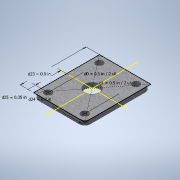
# Autodesk Inventor part: J010354
Saved by Autodesk Inventor 2020.3 (Build 243373000, 373)
## iProperties
RuleStatus: InUse
AfterDocSave0: file://Part Number Cleaner
Created: 2022-03-31
Material: STAINLESS STEEL, 304
Catalog Web Link: https://www.janelia.org/
Vendor: HHMI: JRC - jET
Document SubType Name: Modeling
Designer: arnoldj
Density: 8 g/cm^3
Appearance: Metal-Steel (Stainless, Brushed)
Part Number: J010354
Description: FB CYLINDER PLATE
DESIGN DEPARTMENT: HHMI: JRC - jET
ALTERED ITEM PART NUMBER: N/A
ALTERED ITEM VENDOR: N/A
ALTERED ITEM DESCRIPTION: N/A
Title: Standard
Author: arnoldj
Revision Number: 0
Autodesk Inventor part; units mm, degrees
ref_plane "YZ Plane" through (0, 0, 0) normal (1, 0, 0) x (0, 1, 0)
ref_plane "XZ Plane" through (0, 0, 0) normal (0, 1, 0) x (-1, 0, 0)
ref_plane "XY Plane" through (0, 0, 0) normal (0, 0, 1) x (1, 0, 0)
sketch "Sketch1" plane through (0, 0, 0) normal (0, 1, 0) x (-1, 0, 0)
  line L0 (0, -16.002) -> (0, 16.002) projected
  line L1 (-12.446, 0) -> (12.446, 0) projected
  line L2 (-8.89, 11.43) -> (8.89, 11.43)
  line L3 (8.89, 11.43) -> (8.89, -11.43)
  line L4 (8.89, -11.43) -> (-8.89, -11.43)
  line L5 (-8.89, -11.43) -> (-8.89, 11.43)
  line L6 (-8.89, 11.43) -> (8.89, -11.43) construction
  line L7 (8.89, 11.43) -> (-8.89, -11.43) construction
  point P0 (0, 0)
  point P1 (6.35, 8.89)
  point P2 (-6.35, 8.89)
  dimension "d0" = 6.35
  dimension "d1" = 6.35
  dimension "d23" = 22.86
  dimension "d24" = 17.78
  dimension "d25" = 8.89
  constraints: 12 end point, 2 midpoint, 2 parallel, 1 horizontal, 1 horizontal alignment, 1 perpendicular
  measures "d0" distance from line of L0 point (6.35, 8.89)
  measures "d1" distance from line of L0 point (-6.35, 8.89)
  measures "d23" distance of L2.end L3.end
  measures "d24" distance of L2.start L2.end
  measures "d25" distance from line of L1 point (6.35, 8.89)
extrude "Extrusion1" add sketch "Sketch1" against normal blind 1.524
hole "Hole1" at (-6.35, 0, 8.89) at (6.35, 0, 8.89) direction (0, -1, 0) diameter 2.4384 end through all clearance for "Socket Head Cap Screw" size "#2" standard "Ansi Unified Screw Threads"
sketch "Sketch2" plane through (0, -1.524, 0) normal (0, -1, 0) x (1, 0, 0)
  line L0 (0, 16.002) -> (0, -16.002) projected
  line L1 (-12.446, 0) -> (12.446, 0) projected
  line L2 (-6.477, -4.064) -> (6.477, -4.064)
  line L3 (6.477, -4.064) -> (6.477, 4.064)
  line L4 (6.477, 4.064) -> (-6.477, 4.064)
  line L5 (-6.477, 4.064) -> (-6.477, -4.064)
  line L6 (-6.477, -4.064) -> (6.477, 4.064) construction
  line L7 (6.477, -4.064) -> (-6.477, 4.064) construction
  point P0 (0, 0)
  dimension "d11" = 12.954
  dimension "d12" = 8.128
  constraints: 12 end point, 2 midpoint, 2 parallel, 1 horizontal, 1 perpendicular
  measures "d11" distance of L3.end L4.end
  measures "d12" distance of L4.end L2.start
extrude "Extrusion2" [suppressed]
hole "Hole2" at (0, 0, 0) direction (0, -1, 0) diameter 5.1054 end through all clearance for "Socket Head Cap Screw" size "#10" standard "Ansi Unified Screw Threads"
fillet "Fillet1" radius 1.905 4 edges at (-8.89, -0.762, -11.43) (-8.89, -0.762, 11.43) (8.89, -0.762, 11.43) (8.89, -0.762, -11.43)
mirror "Mirror1" about plane through (0, 0, 0) normal (0, 0, 1) of "Hole1"
body "Solid1"
